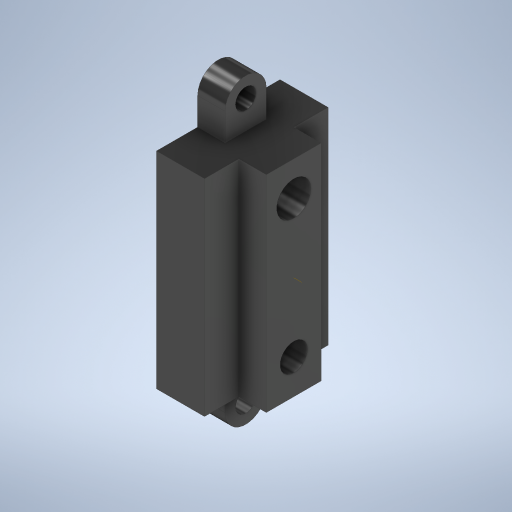
# Autodesk Inventor part: InfraSensor
Saved by Autodesk Inventor 2023 (Build 270158000, 158)
## iProperties
Created: 2024-03-06
Part Number: InfraSensor
Material: Generisch
Document SubType Name: Modeling
Designer: phili
Density: 1 g/cm^3
Appearance: Vorgabe
Author: phili
Autodesk Inventor part; units mm, degrees
ref_plane "YZ Plane" through (0, 0, 0) normal (1, 0, 0) x (0, 1, 0)
ref_plane "XZ Plane" through (0, 0, 0) normal (0, 1, 0) x (-1, 0, 0)
ref_plane "XY Plane" through (0, 0, 0) normal (0, 0, 1) x (1, 0, 0)
sketch "Skizze1" plane through (0, 0, 0) normal (1, 0, 0) x (0, 1, 0)
  line L0 (-15, -9) -> (15, -9)
  line L1 (15, -9) -> (15, 9)
  line L2 (15, 9) -> (-15, 9)
  line L3 (-15, 9) -> (-15, -9)
  line L4 (-15, -9) -> (15, 9) construction
  line L5 (15, -9) -> (-15, 9) construction
  point P0 (0, 0)
  dimension "d0" = 30
  dimension "d1" = 18
  constraints: 12 end point, 2 midpoint, 2 parallel, 1 horizontal, 1 perpendicular
  measures "d0" distance of L2.end L1.end
  measures "d1" distance of L1.end L0.end
extrude "Extrusion1" add sketch "Skizze1" along normal blind 7
sketch "Skizze2" plane through (7, 0, 0) normal (1, 0, 0) x (0, 0, -1)
  line L0 (4, -15) -> (-4, -15)
  line L1 (-4, -15) -> (-4, 15)
  line L2 (-4, 15) -> (4, 15)
  line L3 (4, 15) -> (4, -15)
  line L4 (4, -15) -> (-4, 15) construction
  line L5 (-4, -15) -> (4, 15) construction
  point P0 (0, 0)
  dimension "d4" = 8
  dimension "d5" = 30
  constraints: 12 end point, 2 midpoint, 2 parallel, 1 horizontal, 1 perpendicular
  measures "d4" distance of L1.end L2.end
  measures "d5" distance of L0.end L1.end
extrude "Extrusion2" add sketch "Skizze2" along normal blind 4
sketch "Skizze3" plane through (11, 0, 0) normal (1, 0, 0) x (0, 0, -1)
  point P0 (0, 0)
  point P1 (0.0058, 10)
  dimension "d24" = 10
  measures "d24" distance of point (0, 0) point (0.006, 10)
hole "Bohrung1" at (11, 10, -0.0058) direction (-1, 0, 0) diameter 5 depth 4 tip angle 118
sketch "Skizze4" plane through (11, 0, 0) normal (1, 0, 0) x (0, 0, -1)
  line L0 (-4, -15) -> (4, -15) projected
  point P0 (0, 0)
  point P1 (0, -10)
  dimension "d22" = 0
  dimension "d23" = 5
  measures "d22" horizontal distance of point (0, 0) point (0, -10)
  measures "d23" distance from line of point (0, -10) L0
hole "Bohrung2" at (11, -10, 0) direction (-1, 0, 0) diameter 4 depth 4 tip angle 118
sketch "Skizze5" plane through (0, 0, 0) normal (-1, 0, 0) x (0, 0, 1)
  line L0 (-9, 15) -> (9, 15) projected
  line L1 (-3, 15) -> (-3, 19)
  line L2 (-3, 15) -> (1, 15) construction
  line L3 (3, 15) -> (3, 19)
  line L4 (-3, 15) -> (3, 15)
  arc A0 (3, 19) -> (-3, 19) centre (0, 19) ccw
  point P0 (0, 0)
  point P1 (-3, 17)
  dimension "d25" = 4
  dimension "d26" = 90
  dimension "d27" = 3
  dimension "d28" = 3
  constraints: 8 end point, 2 perpendicular, 2 point on circle, 2 point on line, 2 tangent, 1 centre point, 1 collinear, 1 horizontal, 1 midpoint, 1 vertical
  measures "d25" distance of L1.start L1.end
  measures "d26" angle of L2 L1
  measures "d27" horizontal distance of point (0, 0) point (-3, 17)
  measures "d28" distance from line of point (0, 0) L3
extrude "Extrusion3" add sketch "Skizze5" against normal blind 4
sketch "Skizze6" plane through (4, 0, 0) normal (1, 0, 0) x (0, 0, -1)
  point P0 (0, 0)
  point P1 (0, 19.1025)
  dimension "d38" = 0
  measures "d38" horizontal distance of point (0, 0) point (0, 19.103)
hole "Bohrung3" at (4, 19.1025, 0) direction (-1, 0, 0) diameter 3 depth 4 tip angle 118
mirror "Spiegeln1" about plane through (0, 0, 0) normal (0, 1, 0) of "Extrusion3", "Bohrung3"
